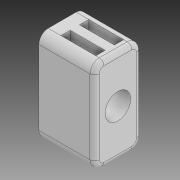
# Autodesk Inventor part: ZBeltBlock
Saved by Autodesk Inventor 2020 (Build 240168000, 168)
## iProperties
Created: 2020-10-26
Part Number: ZBeltBlock
Material: Generic
Document SubType Name: Modeling
Designer: DDeGo
Density: 1 g/cm^3
Appearance: Default
Author: DDeGo
Autodesk Inventor part; units mm, degrees
ref_plane "YZ Plane" through (0, 0, 0) normal (1, 0, 0) x (0, 1, 0)
ref_plane "XZ Plane" through (0, 0, 0) normal (0, 1, 0) x (-1, 0, 0)
sketch "Sketch1" plane through (0, 0, 0) normal (1, 0, 0) x (0, 1, 0)
  line L0 (-10, 5) -> (10, 5)
  line L1 (10, 5) -> (10, -5)
  line L2 (10, -5) -> (-10, -5)
  line L3 (-10, -5) -> (-10, 5)
  line L4 (-10, 5) -> (10, -5) construction
  line L5 (10, 5) -> (-10, -5) construction
  point P0 (0, 0)
  dimension "d0" = 20
  dimension "d1" = 10
  constraints: 12 end point, 2 midpoint, 2 parallel, 1 horizontal, 1 perpendicular
  measures "d0" distance of L1.end L2.end
  measures "d1" distance of L0.end L1.end
extrude "Extrusion1" add sketch "Sketch1" along normal blind 12
sketch "Sketch2" plane through (12, 0, 0) normal (1, 0, 0) x (0, 0, -1)
  circle A0 centre (0, 0) radius 2.75
  line L0 (0, 0) -> (0, 0) construction
  dimension "d4" = 5.5
  dimension "d5" = 0
  constraints: 2 end point, 1 centre point, 1 horizontal
  measures "d4" diameter of A0
  measures "d5" distance of L0.end L0.start
extrude "Extrusion2" cut sketch "Sketch2" against normal through all
ref_plane "Work Plane1" through (6.5, 0, 0) normal (-1, 0, 0) x (0, 0, 1)
sketch "Sketch3" plane through (6.5, 0, 0) normal (-1, 0, 0) x (0, 0, 1)
  line L0 (0, 12.5) -> (0, 7.5) construction
  line L1 (-5, 10) -> (5, 10) projected
  line L2 (1, 12.5) -> (1, 7.5)
  line L3 (-1, 7.5) -> (-1, 12.5)
  arc A0 (1, 12.5) -> (-1, 12.5) centre (0, 12.5) ccw
  arc A1 (-1, 7.5) -> (1, 7.5) centre (0, 7.5) ccw
  line L4 (3, 7.5) -> (3, 12.5)
  arc A2 (3, 12.5) -> (-3, 12.5) centre (0, 12.5) ccw
  line L5 (-3, 12.5) -> (-3, 7.5)
  arc A3 (-3, 7.5) -> (3, 7.5) centre (0, 7.5) ccw
  point P0 (0, 0)
  point P1 (0, 10)
  point P2 (-1, 10)
  point P3 (-3, 10)
  point P4 (3, 10)
  point P5 (1, 10)
  dimension "d9" = 2
  dimension "d10" = 2
  dimension "d11" = 5
  constraints: 12 end point, 8 point on circle, 4 centre point, 4 tangent, 2 midpoint, 2 parallel, 1 perpendicular, 3 other
  measures "d9" distance between parallel lines of L2 L4
  measures "d10" distance between parallel lines of L3 L2
  measures "d11" distance of L0.start L0.end
extrude "Extrusion3" cut sketch "Sketch3" against normal mid plane 7.5 contours L1 L3 A1 L2 L4 A3 L5
mirror "Mirror1" about plane through (0, 0, 0) normal (0, 1, 0) of "Extrusion3"
fillet "Fillet1" radius 2 4 edges at (6, 10, 5) (6, 10, -5) (6, -10, 5) (6, -10, -5)
fillet "Fillet2" radius 1 8 edges at (12, -9.4142, 4.4142) (12, -10, 0) (12, -9.4142, -4.4142) (12, 0, -5) (12, 9.4142, -4.4142) (12, 10, 0) (12, 9.4142, 4.4142) (12, 0, 5)
ref_plane "Work Plane2" through (0, 0, 0) normal (0, 1, 0) x (-1, 0, 0)
body "Solid1"
